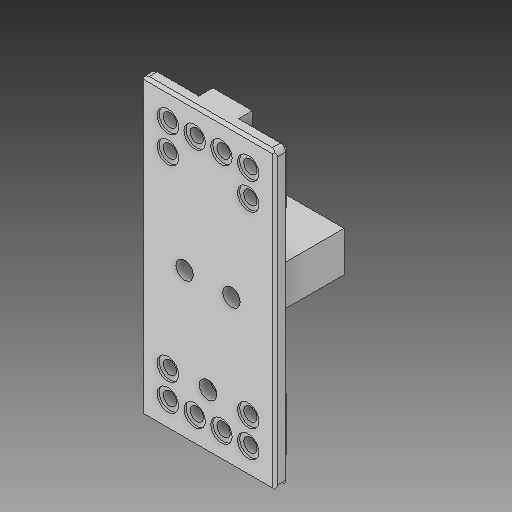
# Autodesk Inventor part: Motor cover upper
Saved by Autodesk Inventor 2019 (Build 230136000, 136)
## iProperties
Created: 2018-12-04
Part Number: Motor cover upper
Material: Generic
Document SubType Name: Modeling
Designer: Varga Daniel
Density: 1 g/cm^3
Appearance: Default
Author: Varga Daniel
Autodesk Inventor part; units mm, degrees
ref_plane "YZ Plane" through (0, 0, 0) normal (1, 0, 0) x (0, 1, 0)
ref_plane "XZ Plane" through (0, 0, 0) normal (0, 1, 0) x (-1, 0, 0)
ref_plane "XY Plane" through (0, 0, 0) normal (0, 0, 1) x (1, 0, 0)
sketch "Sketch1" plane through (0, 0, 0) normal (0, 0, 1) x (1, 0, 0)
  line L0 (13.75, 49.8) -> (-36.25, 49.8)
  line L1 (-36.25, 49.8) -> (-36.25, -60.2)
  line L2 (-36.25, -60.2) -> (13.75, -60.2)
  line L3 (13.75, -60.2) -> (13.75, 49.8)
  circle A0 centre (-2.5, -5.2) radius 2.5 construction
  circle A1 centre (-20, -5.2) radius 2.5 construction
  circle A2 centre (-11.25, -39.5) radius 2.5 construction
  circle A3 centre (-2.5, -5.2) radius 3.25
  circle A4 centre (-20, -5.2) radius 3.25
  circle A5 centre (-11.25, -39.5) radius 3.25
  circle A6 centre (3.75, 29.8) radius 4 construction
  circle A7 centre (-16.25, -50.2) radius 4 construction
  circle A8 centre (3.75, -50.2) radius 4 construction
  circle A9 centre (-16.25, 39.8) radius 4 construction
  circle A10 centre (3.75, 39.8) radius 4 construction
  circle A11 centre (-6.25, 39.8) radius 4 construction
  circle A12 centre (-26.25, 39.8) radius 4 construction
  circle A13 centre (-6.25, -50.2) radius 4 construction
  circle A14 centre (-26.25, -50.2) radius 4 construction
  circle A15 centre (-26.25, 29.8) radius 4 construction
  line L4 (-23.1, -3.4102) -> (-23.1, -6.9898) construction
  line L5 (-23.1, -6.9898) -> (-20, -8.7796) construction
  line L6 (-20, -8.7796) -> (-16.9, -6.9898) construction
  line L7 (-16.9, -6.9898) -> (-16.9, -3.4102) construction
  line L8 (-16.9, -3.4102) -> (-20, -1.6204) construction
  line L9 (-20, -1.6204) -> (-23.1, -3.4102) construction
  line L10 (-5.6, -3.4102) -> (-5.6, -6.9898) construction
  line L11 (-5.6, -6.9898) -> (-2.5, -8.7796) construction
  line L12 (-2.5, -8.7796) -> (0.6, -6.9898) construction
  line L13 (0.6, -6.9898) -> (0.6, -3.4102) construction
  line L14 (0.6, -3.4102) -> (-2.5, -1.6204) construction
  line L15 (-2.5, -1.6204) -> (-5.6, -3.4102) construction
  line L16 (-14.35, -37.7102) -> (-14.35, -41.2898) construction
  line L17 (-14.35, -41.2898) -> (-11.25, -43.0796) construction
  line L18 (-11.25, -43.0796) -> (-8.15, -41.2898) construction
  line L19 (-8.15, -41.2898) -> (-8.15, -37.7102) construction
  line L20 (-8.15, -37.7102) -> (-11.25, -35.9204) construction
  line L21 (-11.25, -35.9204) -> (-14.35, -37.7102) construction
  circle A16 centre (-11.25, -25.8) radius 7.25 construction
  line L22 (-35.25, -59.2) -> (12.75, -59.2) projected
  line L23 (-35.25, 48.8) -> (-35.25, -59.2) projected
  line L24 (12.75, 48.8) -> (-35.25, 48.8) projected
  line L25 (12.75, -59.2) -> (12.75, 48.8) projected
  point P0 (0, 0)
  dimension "d0" = 6.5
  dimension "d1" = 6.5
  dimension "d2" = 6.5
  constraints: 8 end point, 3 centre point, 3 coincident, 2 parallel, 1 horizontal, 1 perpendicular
  measures "d0" diameter of A3
  measures "d1" diameter of A4
  measures "d2" diameter of A5
extrude "Extrusion1" add sketch "Sketch1" along normal blind 4 contours L3 L2 L1 L0 | L23 L24 L25 L22
sketch "Sketch2" plane through (0, 0, 4) normal (0, 0, 1) x (1, 0, 0)
  circle A0 centre (-11.25, -39.5) radius 3.25 construction
  circle A1 centre (-20, -5.2) radius 3.25 construction
  circle A2 centre (-2.5, -5.2) radius 3.25 construction
  line L0 (13.75, 49.8) -> (-36.25, 49.8) construction
  line L1 (-36.25, 49.8) -> (-36.25, -60.2) construction
  line L2 (-36.25, -60.2) -> (13.75, -60.2) construction
  line L3 (13.75, -60.2) -> (13.75, 49.8) construction
  circle A3 centre (-26.25, 39.8) radius 4
  circle A4 centre (-16.25, 39.8) radius 4
  circle A5 centre (-6.25, 39.8) radius 4
  circle A6 centre (3.75, 39.8) radius 4
  circle A7 centre (-26.25, 29.8) radius 4
  circle A8 centre (3.75, 29.8) radius 4
  circle A9 centre (3.75, -50.2) radius 4
  circle A10 centre (-6.25, -50.2) radius 4
  circle A11 centre (-16.25, -50.2) radius 4
  circle A12 centre (-26.25, -50.2) radius 4
  circle A13 centre (-26.25, -40.2) radius 4
  circle A14 centre (3.75, -40.2) radius 4
  point P0 (0, 0)
  dimension "d5" = 8
  dimension "d6" = 10
  dimension "d7" = 10
  dimension "d10" = 10
  dimension "d17" = 10
  dimension "d24" = 10
  dimension "d29" = 8
  dimension "d30" = 10
  dimension "d31" = 10
  dimension "d34" = 10
  dimension "d41" = 10
  dimension "d48" = 10
  constraints: 12 centre point, 4 vertical, 2 horizontal, 20 other
  measures "d5" diameter of A3
  measures "d6" distance from line of A3.centre L1
  measures "d7" distance from line of A3.centre L0
  measures "d10" distance of A3.centre A4.centre
  measures "d17" distance of A3.centre A7.centre
  measures "d24" distance of A6.centre A8.centre
  measures "d29" diameter of A9
  measures "d30" distance from line of A9.centre L3
  measures "d31" distance from line of A9.centre L2
  measures "d34" distance of A9.centre A10.centre
  measures "d41" distance of A12.centre A13.centre
  measures "d48" distance of A9.centre A14.centre
extrude "Extrusion2" cut sketch "Sketch2" against normal blind 0.8
sketch "Sketch3" plane through (0, 0, 0) normal (0, 0, -1) x (-1, 0, 0)
  circle A0 centre (11.25, -39.5) radius 3.25 construction
  circle A1 centre (20, -5.2) radius 3.25 construction
  circle A2 centre (2.5, -5.2) radius 3.25 construction
  line L0 (-13.75, 49.8) -> (36.25, 49.8) construction
  line L1 (-13.75, -60.2) -> (-13.75, 49.8) construction
  line L2 (36.25, -60.2) -> (-13.75, -60.2) construction
  line L3 (36.25, 49.8) -> (36.25, -60.2) construction
  line L4 (31.25, 44.8) -> (-8.75, 44.8)
  line L5 (-8.75, 44.8) -> (-8.75, -55.2)
  line L6 (-8.75, -55.2) -> (31.25, -55.2)
  line L7 (31.25, -55.2) -> (31.25, 44.8)
  line L8 (31.25, 44.8) -> (-8.75, 44.8)
  line L9 (-8.75, 44.8) -> (-8.75, 34.8)
  line L10 (-8.75, 34.8) -> (31.25, 34.8)
  line L11 (31.25, 34.8) -> (31.25, 44.8)
  line L12 (31.25, -55.2) -> (-8.75, -55.2)
  line L13 (-8.75, -55.2) -> (-8.75, -45.2)
  line L14 (-8.75, -45.2) -> (31.25, -45.2)
  line L15 (31.25, -45.2) -> (31.25, -55.2)
  line L16 (31.25, 34.8) -> (21.25, 34.8)
  line L17 (21.25, 34.8) -> (21.25, 24.8)
  line L18 (21.25, 24.8) -> (31.25, 24.8)
  line L19 (31.25, 24.8) -> (31.25, 34.8)
  line L20 (-8.75, 34.8) -> (1.25, 34.8)
  line L21 (1.25, 34.8) -> (1.25, 24.8)
  line L22 (1.25, 24.8) -> (-8.75, 24.8)
  line L23 (-8.75, 24.8) -> (-8.75, 34.8)
  line L24 (31.25, -45.2) -> (21.25, -45.2)
  line L25 (21.25, -45.2) -> (21.25, -35.2)
  line L26 (21.25, -35.2) -> (31.25, -35.2)
  line L27 (31.25, -35.2) -> (31.25, -45.2)
  line L28 (-8.75, -45.2) -> (1.25, -45.2)
  line L29 (1.25, -45.2) -> (1.25, -35.2)
  line L30 (1.25, -35.2) -> (-8.75, -35.2)
  line L31 (-8.75, -35.2) -> (-8.75, -45.2)
  point P0 (0, 0)
  dimension "d55" = 5
  dimension "d56" = 5
  dimension "d57" = 5
  dimension "d58" = 5
  dimension "d59" = 10
  dimension "d60" = 10
  dimension "d70" = 10
  dimension "d71" = 10
  dimension "d72" = 10
  dimension "d73" = 10
  dimension "d74" = 10
  dimension "d75" = 10
  dimension "d76" = 10
  dimension "d77" = 10
  constraints: 56 end point, 14 parallel, 7 horizontal, 7 perpendicular, 2 point on line
  measures "d55" distance between parallel lines of L2 L6
  measures "d56" distance between parallel lines of L7 L3
  measures "d57" distance between parallel lines of L1 L5
  measures "d58" distance between parallel lines of L0 L4
  measures "d59" distance between parallel lines of L4 L10
  measures "d60" distance between parallel lines of L14 L6
  measures "d70" distance of L18.end L17.end
  measures "d71" distance of L17.end L16.end
  measures "d72" distance of L21.end L22.end
  measures "d73" distance of L20.end L21.end
  measures "d74" distance of L25.end L26.end
  measures "d75" distance of L24.end L25.end
  measures "d76" distance of L30.end L29.end
  measures "d77" distance of L29.end L28.end
extrude "Extrusion3" add sketch "Sketch3" along normal blind 5.2 contours L7 L10 L5 L4 | L7 L18 L17 L10 | L10 L21 L22 L5 | L7 L14 L25 L26 | L30 L29 L14 L5 | L7 L6 L5 L14
sketch "Sketch4" plane through (0, 0, 4) normal (0, 0, 1) x (1, 0, 0)
  circle A0 centre (-26.25, -40.2) radius 4 construction
  circle A1 centre (-16.25, -50.2) radius 4 construction
  circle A2 centre (3.75, -50.2) radius 4 construction
  circle A3 centre (-26.25, 29.8) radius 4 construction
  circle A4 centre (-6.25, 39.8) radius 4 construction
  circle A5 centre (-26.25, 39.8) radius 4 construction
  circle A6 centre (-16.25, 39.8) radius 4 construction
  circle A7 centre (3.75, 39.8) radius 4 construction
  circle A8 centre (3.75, 29.8) radius 4 construction
  circle A9 centre (-6.25, -50.2) radius 4 construction
  circle A10 centre (-26.25, -50.2) radius 4 construction
  circle A11 centre (3.75, -40.2) radius 4 construction
  circle A12 centre (-11.25, -39.5) radius 3.25 construction
  circle A13 centre (-20, -5.2) radius 3.25 construction
  circle A14 centre (-2.5, -5.2) radius 3.25 construction
  line L0 (13.75, 49.8) -> (-36.25, 49.8) construction
  line L1 (-36.25, 49.8) -> (-36.25, -60.2) construction
  line L2 (-36.25, -60.2) -> (13.75, -60.2) construction
  line L3 (13.75, -60.2) -> (13.75, 49.8) construction
  point P0 (0, 0)
hole "Hole1" at (-26.25, 39.8, 4) at (-16.25, 39.8, 4) at (-6.25, 39.8, 4) at (3.75, 39.8, 4) at (3.75, 29.8, 4) at (-26.25, 29.8, 4) at (-26.25, -50.2, 4) at (-26.25, -40.2, 4) at (-16.25, -50.2, 4) at (-6.25, -50.2, 4) at (3.75, -50.2, 4) at (3.75, -40.2, 4) direction (0, 0, -1) diameter 5 end through all
sketch "Sketch5" plane through (0, 0, 0) normal (0, 0, -1) x (-1, 0, 0)
  line L0 (-8.75, 44.8) -> (31.25, 44.8) construction
  line L1 (31.25, 44.8) -> (31.25, 24.8) construction
  line L2 (31.25, 24.8) -> (21.25, 24.8) construction
  line L3 (21.25, 24.8) -> (21.25, 34.8) construction
  line L4 (21.25, 34.8) -> (1.25, 34.8) construction
  line L5 (1.25, 34.8) -> (1.25, 24.8) construction
  line L6 (1.25, 24.8) -> (-8.75, 24.8) construction
  line L7 (-8.75, 24.8) -> (-8.75, 44.8) construction
  line L8 (1.25, -45.2) -> (21.25, -45.2) construction
  line L9 (21.25, -45.2) -> (21.25, -35.2) construction
  line L10 (21.25, -35.2) -> (31.25, -35.2) construction
  line L11 (31.25, -35.2) -> (31.25, -55.2) construction
  line L12 (31.25, -55.2) -> (-8.75, -55.2) construction
  line L13 (-8.75, -55.2) -> (-8.75, -35.2) construction
  line L14 (-8.75, -35.2) -> (1.25, -35.2) construction
  line L15 (1.25, -35.2) -> (1.25, -45.2) construction
  circle A0 centre (11.25, -39.5) radius 3.25 construction
  circle A1 centre (20, -5.2) radius 3.25 construction
  circle A2 centre (2.5, -5.2) radius 3.25 construction
  line L16 (-13.75, 49.8) -> (36.25, 49.8) construction
  line L17 (-13.75, -60.2) -> (-13.75, 49.8) construction
  line L18 (36.25, -60.2) -> (-13.75, -60.2) construction
  line L19 (36.25, 49.8) -> (36.25, -60.2) construction
  line L20 (-13.75, 49.8) -> (36.25, 49.8) construction
  line L21 (11.25, 49.8) -> (11.25, 44.8) construction
  line L22 (3.85, 49.8) -> (18.65, 49.8)
  line L23 (18.65, 49.8) -> (18.65, 44.8)
  line L24 (18.65, 44.8) -> (3.85, 44.8)
  line L25 (3.85, 44.8) -> (3.85, 49.8)
  point P0 (0, 0)
  dimension "d78" = 14.8
  constraints: 10 end point, 2 midpoint, 2 parallel, 2 point on line, 1 horizontal, 1 perpendicular, 1 other
  measures "d78" distance between parallel lines of L23 L25
extrude "Extrusion4" add sketch "Sketch5" along normal up to surface (5.2 mm away)
chamfer "Chamfer1" distance 1 angle 45 4 edges at (13.75, -5.2, 4) (-11.25, 49.8, 4) (-36.25, -5.2, 4) (-11.25, -60.2, 4)
fillet "Fillet1" radius 2 4 edges at (13.75, 49.8, 1.5) (-36.25, 49.8, 1.5) (13.75, -60.2, 1.5) (-36.25, -60.2, 1.5)
sketch "Sketch6" plane through (0, 0, 0) normal (0, 0, -1) x (-1, 0, 0)
  line L0 (-3.75, 2.3) -> (26.25, 2.3)
  line L1 (26.25, 2.3) -> (26.25, -12.7)
  line L2 (26.25, -12.7) -> (-3.75, -12.7)
  line L3 (-3.75, -12.7) -> (-3.75, 2.3)
  circle A0 centre (2.5, -5.2) radius 3.25 construction
  circle A1 centre (20, -5.2) radius 3.25 construction
  circle A2 centre (11.25, -39.5) radius 3.25 construction
  line L4 (1.25, -45.2) -> (21.25, -45.2) construction
  line L5 (21.25, -45.2) -> (21.25, -35.2) construction
  line L6 (21.25, -35.2) -> (31.25, -35.2) construction
  line L7 (31.25, -35.2) -> (31.25, -55.2) construction
  line L8 (31.25, -55.2) -> (-8.75, -55.2) construction
  line L9 (-8.75, -55.2) -> (-8.75, -35.2) construction
  line L10 (-8.75, -35.2) -> (1.25, -35.2) construction
  line L11 (1.25, -35.2) -> (1.25, -45.2) construction
  arc A3 (34.25, -60.2) -> (36.25, -58.2) centre (34.25, -58.2) ccw construction
  line L12 (36.25, 47.8) -> (36.25, -58.2) construction
  arc A4 (36.25, 47.8) -> (34.25, 49.8) centre (34.25, 47.8) ccw construction
  line L13 (18.65, 49.8) -> (34.25, 49.8) construction
  line L14 (18.65, 49.8) -> (18.65, 44.8) construction
  line L15 (18.65, 44.8) -> (31.25, 44.8) construction
  line L16 (31.25, 44.8) -> (31.25, 24.8) construction
  line L17 (31.25, 24.8) -> (21.25, 24.8) construction
  line L18 (21.25, 24.8) -> (21.25, 34.8) construction
  line L19 (21.25, 34.8) -> (1.25, 34.8) construction
  line L20 (1.25, 34.8) -> (1.25, 24.8) construction
  line L21 (1.25, 24.8) -> (-8.75, 24.8) construction
  line L22 (-8.75, 24.8) -> (-8.75, 44.8) construction
  line L23 (-8.75, 44.8) -> (3.85, 44.8) construction
  line L24 (3.85, 44.8) -> (3.85, 49.8) construction
  line L25 (-11.75, 49.8) -> (3.85, 49.8) construction
  arc A5 (-11.75, 49.8) -> (-13.75, 47.8) centre (-11.75, 47.8) ccw construction
  line L26 (-13.75, -58.2) -> (-13.75, 47.8) construction
  arc A6 (-13.75, -58.2) -> (-11.75, -60.2) centre (-11.75, -58.2) ccw construction
  line L27 (34.25, -60.2) -> (-11.75, -60.2) construction
  line L28 (3.5982, -5.2) -> (20, -5.2) construction
  line L29 (34.25, -60.2) -> (-11.75, -60.2) construction
  line L30 (11.25, -60.2) -> (11.25, -26.9052) construction
  circle A7 centre (2.5, -5.2) radius 1.35
  circle A8 centre (20, -5.2) radius 1.35
  point P0 (0, 0)
  dimension "d85" = 15
  dimension "d86" = 30
  dimension "d89" = 2.7
  dimension "d90" = 2.7
  constraints: 12 end point, 2 centre point, 2 coincident, 2 horizontal, 2 parallel, 2 perpendicular, 1 midpoint, 2 other
  measures "d85" distance between parallel lines of L2 L0
  measures "d86" distance between parallel lines of L1 L3
  measures "d89" diameter of A7
  measures "d90" diameter of A8
ref_plane "Work Plane1" through (-22.2, -36.7, -31.9) normal (0, 0, 1) x (1, 0, 0)
extrude "Extrusion6" add sketch "Sketch6" along normal blind 31.8
sketch "Sketch7" plane through (-2.5, -5.2, 0) normal (0, 0, 1) x (1, 0, 0)
  circle A0 centre (0, 0) radius 3.25 projected
  circle A1 centre (-17.5, 0) radius 3.25 projected
  point P0 (2.5, 5.2)
extrude "Extrusion7" cut sketch "Sketch7" against normal blind 26
equation "\"d56\" = d55"
equation "\"d57\" = d55"
equation "\"d58\" = d55"
body "Solid1"
